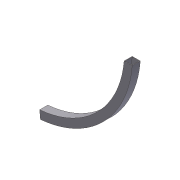
# Autodesk Inventor part: Shooter_Frame_RearGuide
Saved by Autodesk Inventor 2012 (Build 160160000, 160)
## iProperties
Created: 2012-01-18
Part Number: Shooter_Frame_RearGuide
Material: Aluminum-6061
Document SubType Name: Modeling
Designer: JesseK
Mass: 174.848 g
Surface Area: 815.873 cm^2
Volume: 64.5194 cm^3
Density: 2.71 g/cm^3
Author: JesseK
Autodesk Inventor part; units mm, degrees
ref_plane "YZ Plane" through (0, 0, 0) normal (1, 0, 0) x (0, 1, 0)
ref_plane "XZ Plane" through (0, 0, 0) normal (0, 1, 0) x (-1, 0, 0)
ref_plane "XY Plane" through (0, 0, 0) normal (0, 0, 1) x (1, 0, 0)
sketch "Sketch1" plane through (0, 0, 0) normal (0, 0, 1) x (1, 0, 0)
  arc A0 (25.5164, -290.9834) -> (290.9936, -25.4) centre (0, 0) ccw
  arc A1 (27.7352, -316.2863) -> (316.4824, -25.4) centre (0, 0) ccw
  line L0 (25.5164, -290.9834) -> (27.7352, -316.2863)
  line L1 (290.9936, -25.4) -> (316.4824, -25.4)
  line L2 (0, 0) -> (25.5164, -290.9834) construction
  line L3 (0, -292.1) -> (0, 0) construction
  line L4 (290.9936, -25.4) -> (0, 0) construction
  line L5 (290.9936, 0) -> (316.4824, 0) construction
  line L6 (316.4824, 0) -> (316.4824, -25.4) construction
  line L7 (316.4824, -25.4) -> (290.9936, -25.4) construction
  line L8 (290.9936, -25.4) -> (290.9936, 0) construction
  line L9 (0, 0) -> (359.7285, 0) construction
  dimension "d0" = 292.1
  dimension "d1" = 25.4
  dimension "d9" = 25.4
  dimension "d10" = 80
  constraints: 21 end point, 4 point on circle, 3 coincident, 2 centre point, 2 horizontal, 2 parallel, 1 collinear, 1 perpendicular, 1 point on line, 1 vertical
  measures "d0" radius of A0
  measures "d1" radial gap between concentric circles of A1 A0
  measures "d9" distance of L1.start L5.start
  measures "d10" angle of L2 L4
extrude "Extrusion1" add sketch "Sketch1" along normal blind 25.4
shell "Shell1" thickness 1.5875 removed faces 2 at (299.4898, -25.4, 8.4667) at (26.9956, -307.852, 16.9333)
body "Solid1"
